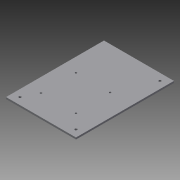
# Autodesk Inventor part: bottomLayer
Saved by Autodesk Inventor 2014 (Build 180170000, 170)
## iProperties
Created: 2014-11-25
Part Number: bottomLayer
Material: Generic
Document SubType Name: Modeling
Designer: Rachel
Density: 1 g/cm^3
Appearance: Default
Author: Rachel
Autodesk Inventor part; units mm, degrees
ref_plane "YZ Plane" through (0, 0, 0) normal (1, 0, 0) x (0, 1, 0)
ref_plane "XZ Plane" through (0, 0, 0) normal (0, 1, 0) x (-1, 0, 0)
ref_plane "XY Plane" through (0, 0, 0) normal (0, 0, 1) x (1, 0, 0)
sketch "Base" plane through (0, 0, 0) normal (0, 1, 0) x (-1, 0, 0)
  line L0 (0, 0) -> (127, 0)
  line L1 (127, 0) -> (127, 177.8)
  line L2 (127, 177.8) -> (0, 177.8)
  line L3 (0, 177.8) -> (0, 0)
  dimension "d7" = 127
  dimension "d8" = 177.8
  constraints: 8 end point, 2 parallel, 1 horizontal, 1 perpendicular
  measures "d7" distance of L2.end L1.end
  measures "d8" distance of L1.end L0.end
extrude "Base 1/8\"" add sketch "Base" along normal blind 3.175
sketch "TopLayer" plane through (0, 3.175, 0) normal (0, 1, 0) x (1, 0, 0)
  point P0 (-114.3, -165.1)
  point P1 (-12.7, -165.1)
  point P2 (-12.7, -12.7)
hole "TopLayerHoles" at (-114.3, 3.175, 165.1) at (-12.7, 3.175, 165.1) at (-12.7, 3.175, 12.7) direction (0, -1, 0) diameter 4.191 end through all
sketch "Controller" plane through (0, 3.175, 0) normal (0, 1, 0) x (1, 0, 0)
  line L0 (0, 0) -> (-127, 0) projected
  line L1 (-127, 0) -> (-127, -177.8) projected
  line L2 (-127, -152.4) -> (-25.4, -152.4) construction
  line L3 (-127, -152.4) -> (-25.4, -152.4) construction
  line L4 (-25.4, -152.4) -> (-25.4, 0) construction
  line L5 (-140.6178, -177.8) -> (-108.8678, -177.8) construction
  line L6 (-31.75, -146.05) -> (-107.95, -146.05) construction
  line L7 (-107.95, -146.05) -> (-107.95, -69.85) construction
  line L8 (-107.95, -69.85) -> (-31.75, -69.85) construction
  line L9 (-31.75, -69.85) -> (-31.75, -146.05) construction
  line L10 (-31.75, -146.05) -> (-38.1, -146.05) construction
  line L11 (-38.1, -146.05) -> (-38.1, -139.7) construction
  line L12 (-38.1, -139.7) -> (-31.75, -139.7) construction
  line L13 (-31.75, -139.7) -> (-31.75, -146.05) construction
  line L14 (-107.95, -69.85) -> (-101.6, -69.85) construction
  line L15 (-101.6, -69.85) -> (-101.6, -76.2) construction
  line L16 (-101.6, -76.2) -> (-107.95, -76.2) construction
  line L17 (-107.95, -76.2) -> (-107.95, -69.85) construction
  circle A0 centre (-38.1, -139.7) radius 1.651
  circle A1 centre (-101.6, -139.7) radius 1.651
  circle A2 centre (-101.6, -76.2) radius 1.651
  circle A3 centre (-39.751, -76.2) radius 1.651
  dimension "d36" = 76.2
  dimension "d37" = 76.2
  dimension "d38" = 6.35
  dimension "d39" = 6.35
  dimension "d40" = 6.35
  dimension "d41" = 6.35
  dimension "d42" = 3.302
  dimension "d43" = 3.302
  dimension "d44" = 3.302
  dimension "d45" = 3.302
  constraints: 32 end point, 6 coincident, 6 parallel, 5 horizontal, 4 centre point, 4 perpendicular, 2 point on line, 1 collinear
  measures "d36" distance of L7.end L8.end
  measures "d37" distance of L6.end L7.end
  measures "d38" distance of L11.end L12.end
  measures "d39" distance of L10.end L11.end
  measures "d40" distance of L15.end L16.end
  measures "d41" distance of L14.end L15.end
  measures "d42" diameter of A0
  measures "d43" diameter of A1
  measures "d44" diameter of A2
  measures "d45" diameter of A3
hole "ControllerHoles" at (-38.1, 3.175, 139.7) at (-39.751, 3.175, 76.2) at (-101.6, 3.175, 76.2) at (-101.6, 3.175, 139.7) direction (0, -1, 0) diameter 3.302 end through all
body "Solid2"
